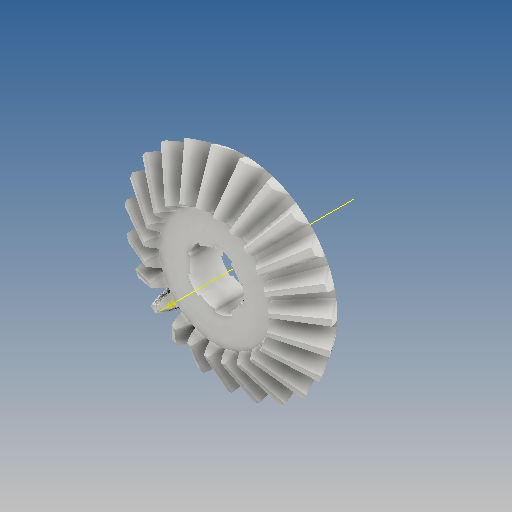
# Autodesk Inventor part: PWTR-0058
Saved by Autodesk Inventor 2021.1 (Build 251245000, 245)
## iProperties
CustomPartVersion: 1
Created: 2020-08-27
Material: Steel, Mild
Document SubType Name: Modeling
Designer: alid
Categories: <?xml version="1.0" encoding="UTF-16"?> <MemberInstance><Categories><FamilyTemplate><FamilyTemplateParameter ValueType="xs:double" Id="1" ObjectReferenceKey="da_z" ObjectType="kUserParameterObject"/><FamilyTemplateParameter ValueType="xs:double" Id="2" ObjectReferenceKey="da_b" ObjectType="kUserParameterObject"/><FamilyTemplateParameter ValueType="xs:double" Id="3" ObjectReferenceKey="da_beta" ObjectType="kUserParameterObject"/><FamilyTemplateParameter ValueType="xs:double" Id="4" ObjectReferenceKey="da_dae" ObjectType="kUserParameterObject"/><FamilyTemplateParameter ValueType="xs:double" Id="5" ObjectReferenceKey="da_ve" ObjectType="kUserParameterObject"/><FamilyTemplateParameter ValueType="xs:double" Id="6" ObjectReferenceKey="da_omega" ObjectType="kUserParameterObject"/><FamilyTemplateParameter ValueType="xs:string" Id="7" ObjectReferenceKey="EAIAABAAAAAAHwAAAAAAAIAAAAAAAAAA" ObjectType="83914240" SubObjectId="SurfaceGeometry"/></FamilyTemplate><ParamToTemplateMap><ParamToTemplate CategoryParameter="//CategoryParameter[@InternalName='046C89C9-8512-4d59-83FE-43B91F4F132A']" TemplateParameter="1"/><ParamToTemplate CategoryParameter="//CategoryParameter[@InternalName='2552DF32-E462-4b46-AEBF-C6C7768E72AC']" TemplateParameter="2"/><ParamToTemplate CategoryParameter="//CategoryParameter[@InternalName='C9EE641D-15FC-4fae-A226-E94C4372FDD7']" TemplateParameter="3"/><ParamToTemplate><ParamToTemplate CategoryParameter="//CategoryParameter[@InternalName='00B6519A-459B-49c7-AD84-2E56D39A5744']" ConstantValue="0.000000"/></ParamToTemplate><ParamToTemplate><ParamToTemplate CategoryParameter="//CategoryParameter[@InternalName='04B31F0E-C7A6-4894-AA32-9629BEFACF47']" ConstantValue="1.000000"/></ParamToTemplate><ParamToTemplate><ParamToTemplate CategoryParameter="//CategoryParameter[@InternalName='43CBEC2E-7847-49e7-A936-2F7889FCB2D9']" ConstantValue="0.200000"/></ParamToTemplate><ParamToTemplate><ParamToTemplate CategoryParameter="//CategoryParameter[@InternalName='B1EFC894-105D-4ebd-86BF-FA20ED196853']" ConstantValue="0.266800"/></ParamToTemplate><ParamToTemplate><ParamToTemplate CategoryParameter="//CategoryParameter[@InternalName='51175063-3D10-4879-93E8-6246FE8B403D']" ConstantValue="2060000000.000000"/></ParamToTemplate><ParamToTemplate><ParamToTemplate CategoryParameter="//CategoryParameter[@InternalName='A3A52E27-4454-46a9-B0BD-C932399B70AF']" ConstantValue="0.300000"/></ParamToTemplate><ParamToTemplate CategoryParameter="//CategoryParameter[@InternalName='2A200944-5A8C-41ca-B96E-8520D2E510F1']" TemplateParameter="4"/><ParamToTemplate><ParamToTemplate CategoryParameter="//CategoryParameter[@InternalName='1A637F62-92C8-44bc-B81F-10802510B579']" ConstantValue="4.349894"/></ParamToTemplate><ParamToTemplate CategoryParameter="//CategoryParameter[@InternalName='B52DD4BE-6863-48fb-BF58-89EF6F9EC65C']" TemplateParameter="5"/><ParamToTemplate><ParamToTemplate CategoryParameter="//CategoryParameter[@InternalName='3956BFF2-84D2-457d-93C2-9B0613DEBA67']" ConstantValue="1.202891"/></ParamToTemplate><ParamToTemplate CategoryParameter="//CategoryParameter[@InternalName='739CFA02-461B-4bf8-8049-181FCAD8B28F']" TemplateParameter="6"/><ParamToTemplate><ParamToTemplate CategoryParameter="//CategoryParameter[@InternalName='A27E999F-E2CE-4481-8A2A-EBF499C4C3C5']" ConstantValue="0.000000"/></ParamToTemplate><ParamToTemplate><ParamToTemplate CategoryParameter="//CategoryParameter[@InternalName='9E1B4470-B2D3-4ff1-B813-535BB4CDF51A']" ConstantValue="3520000.000000"/></ParamToTemplate><ParamToTemplate><ParamToTemplate CategoryParameter="//CategoryParameter[@InternalName='F8452263-BFF6-458c-9FB1-07C4B99E95CD']" ConstantValue="11400000.000000"/></ParamToTemplate><ParamToTemplate><ParamToTemplate CategoryParameter="//CategoryParameter[@InternalName='3E3BB259-FD49-497f-8171-6EBC954A3479']" ConstantValue="2.000000"/></ParamToTemplate><ParamToTemplate CategoryParameter="//CategoryParameter[@InternalName='27C3BAF2-7550-4e4b-AE2C-0DB134B7D9B7']" TemplateParameter="7"/></ParamToTemplateMap><Category DisplayName="Gear" InternalName="DC85795E-93AB-48d5-8EEE-5A27447B64BD" Mnemonic="Gear"><CategoryParameter DisplayName="z" InternalName="046C89C9-8512-4d59-83FE-43B91F4F132A" Mnemonic="z"/><CategoryParameter DisplayName="b" InternalName="2552DF32-E462-4b46-AEBF-C6C7768E72AC" Mnemonic="b"/><CategoryParameter DisplayName="||b|" InternalName="C9EE641D-15FC-4fae-A226-E94C4372FDD7" Mnemonic="beta"/><CategoryParameter DisplayName="x" InternalName="00B6519A-459B-49c7-AD84-2E56D39A5744" Mnemonic="x"/><CategoryParameter DisplayName="a*" InternalName="04B31F0E-C7A6-4894-AA32-9629BEFACF47" Mnemonic="a"/><CategoryParameter DisplayName="c*" InternalName="43CBEC2E-7847-49e7-A936-2F7889FCB2D9" Mnemonic="c"/><CategoryParameter DisplayName="r|.f|*" InternalName="B1EFC894-105D-4ebd-86BF-FA20ED196853" Mnemonic="rf"/><CategoryParameter DisplayName="E" InternalName="51175063-3D10-4879-93E8-6246FE8B403D" Mnemonic="E"/><CategoryParameter DisplayName="||m|" InternalName="A3A52E27-4454-46a9-B0BD-C932399B70AF" Mnemonic="mi"/><Category DisplayName="BevelGear" InternalName="0C98F69A-0C2B-4791-B2FE-7691BB227E77" Mnemonic="BevelGear"><CategoryParameter DisplayName="d|.ae|" InternalName="2A200944-5A8C-41ca-B96E-8520D2E510F1" Mnemonic="dae"/><CategoryParameter DisplayName="d|.ai|" InternalName="1A637F62-92C8-44bc-B81F-10802510B579" Mnemonic="dai"/><CategoryParameter DisplayName="A|.e|" InternalName="B52DD4BE-6863-48fb-BF58-89EF6F9EC65C" Mnemonic="ve"/><CategoryParameter DisplayName="A|.i|" InternalName="3956BFF2-84D2-457d-93C2-9B0613DEBA67" Mnemonic="vi"/><CategoryParameter DisplayName="||S|" InternalName="739CFA02-461B-4bf8-8049-181FCAD8B28F" Mnemonic="omega"/><CategoryParameter DisplayName="x|.t|" InternalName="A27E999F-E2CE-4481-8A2A-EBF499C4C3C5" Mnemonic="xt"/><CategoryParameter DisplayName="||s||.Flim|" InternalName="9E1B4470-B2D3-4ff1-B813-535BB4CDF51A" Mnemonic="sFlim"/><CategoryParameter DisplayName="||s||.Hlim|" InternalName="F8452263-BFF6-458c-9FB1-07C4B99E95CD" Mnemonic="sHlim"/><CategoryParameter DisplayName="type" InternalName="3E3BB259-FD49-497f-8171-6EBC954A3479" Mnemonic="type"/><CategoryParameter DisplayName="PitchDiameter" InternalName="27C3BAF2-7550-4e4b-AE2C-0DB134B7D9B7" Mnemonic="IDS_PITCHDIAM"/></Category></Category></Categories></MemberInstance>
Mass: 60.9118 g
Surface Area: 34.3074 cm^2
Volume: 7.7496 cm^3
Density: 7.86 g/cm^3
Appearance: Steel
Description: Bevel Transfer Gear
Part Number: PWTR-0058
Author: alid
Revision Number: A
Autodesk Inventor part; units mm, degrees
ref_plane "Mesh Plane2" through (0, 0, 0) normal (0.9906859, 0.1361666, 0) x (0, 0, 1)
sketch "Teeth Body Sketch" plane through (0, 0, 0) normal (1, 0, 0) x (0, 1, 0)
  line L0 (0, 0) -> (32.533436, -25.515398) construction
  line L1 (32.533436, -25.515398) -> (36.138803, -19.987168)
  line L2 (36.138803, -19.987168) -> (0, 0) construction
  line L3 (34.5, -22.5) -> (0, 0) construction
  line L4 (19.579646, -15.35597) -> (21.74947, -12.028907)
  line L5 (32.533436, -25.515398) -> (19.579646, -15.35597)
  line L6 (36.138803, -19.987168) -> (21.74947, -12.028907)
  line L7 (0, -24.879989) -> (0, 4.146665)
  line L8 (0, -22.5) -> (36.138803, -22.5) construction
  dimension "d0" = 69
  dimension "d1" = 65.06687
  dimension "d2" = 72.27761
  dimension "d3" = 16.4
  dimension "d4" = 19.98717
  constraints: 16 end point, 4 point on line, 3 perpendicular, 2 collinear, 1 horizontal alignment, 1 vertical alignment
  measures "d0" diameter of L3.start L7
  measures "d1" diameter of L0.end L7
  measures "d2" diameter of L1.end L7
  measures "d3" distance between parallel lines of L1 L4
  measures "d4" vertical distance of L1.end L0.start
revolve "Teeth Body" add sketch "Teeth Body Sketch" angle 360 about axis through (0, 0, 0) along (0, 0, 1)
ref_plane "Tooth Plane" through (0, 34.5, -22.5) normal (0, -0.8376106, 0.5462678) x (1, 0, 0)
sketch "Start Sketch" plane through (0, 34.5, -22.5) normal (0, -0.8376106, 0.5462678) x (1, 0, 0)
  line L0 (0, -39.723332) -> (0, 12.461154)
  arc A0 (-1.111235, -4.392) -> (-5.068702, 4.791205) centre (-23.36018, -8.535768) ccw
  arc A1 (5.068702, 4.791205) -> (1.111235, -4.392) centre (23.36018, -8.535768) ccw
  line L1 (-1.111235, -4.392) -> (1.111235, -4.392)
  arc A2 (5.068702, 4.791205) -> (-5.068702, 4.791205) centre (0, -63.155839) ccw
  dimension "d7" = 22.63154
  dimension "d8" = 23.36018
  dimension "d9" = 54.62007
  dimension "d57" = 68.13584
  dimension "d58" = 58.76384
  constraints: 6 point on circle, 3 centre point, 3 symmetric about line, 2 end point, 1 coincident, 1 perpendicular, 1 other
  measures "d7" radius of A0
  measures "d8" horizontal distance of point (0, -63.156) A0.centre
  measures "d9" vertical distance of point (0, -63.156) A0.centre
  measures "d57" radius of A2
  measures "d58" distance from line of A2.centre L1
sketch "End Sketch" plane through (0, 20.486775, -13.36094) normal (0, -0.8376106, 0.5462678) x (1, 0, 0)
  line L0 (0, -23.451185) -> (0, 7.356604)
  arc A0 (-0.659873, -2.608055) -> (-3.009894, 2.845111) centre (-13.871732, -5.068706) ccw
  arc A1 (3.009894, 2.845111) -> (0.659873, -2.608055) centre (13.871732, -5.068706) ccw
  line L1 (-0.659873, -2.608055) -> (0.659873, -2.608055)
  arc A2 (3.009894, 2.845111) -> (-3.009894, 2.845111) centre (0, -37.503172) ccw
  dimension "d12" = 13.43905
  dimension "d15" = 13.87173
  dimension "d16" = 32.43447
  dimension "d59" = 40.46039
  dimension "d60" = 34.89512
  constraints: 6 point on circle, 3 centre point, 3 symmetric about line, 2 end point, 1 coincident, 1 other
  measures "d12" radius of A0
  measures "d15" horizontal distance of A0.centre point (0, -37.503)
  measures "d16" vertical distance of A0.centre point (0, -37.503)
  measures "d59" radius of A2
  measures "d60" distance from line of A2.centre L1
loft "Loft" cut profiles "Start Sketch", "End Sketch"
pattern_circular "Circular Pattern" count 23 over 360 about axis through (0, 0, 0) along (0, 0, 1) of "Loft"
ref_plane "End Plane" through (0, 20.486775, -13.36094) normal (0, -0.8376106, 0.5462678) x (1, 0, 0)
sketch3d "3D Sketch Right"
ref_plane "End Plane Right" through (-4.87651, 19.897929, -13.36094) normal (0.1993782, -0.8135354, 0.5462678) x (0.9712573, 0.2380321, 0)
sketch "End Sketch Right" plane through (-4.87651, 19.897929, -13.36094) normal (0.1993782, -0.8135354, 0.5462678) x (0.9712573, 0.2380321, 0)
  arc A0 (-0.659873, -2.608055) -> (-3.009894, 2.845111) centre (-13.871732, -5.068706) ccw
  line L0 (0, -48.37326) -> (0, 13.825579)
  arc A1 (3.009894, 2.845111) -> (0.659873, -2.608055) centre (13.871732, -5.068706) ccw
  line L1 (-0.659873, -2.608055) -> (0.659873, -2.608055)
  arc A2 (3.009894, 2.845111) -> (-3.009894, 2.845111) centre (0, -37.503172) ccw
  dimension "d70" = 13.87173
  dimension "d71" = 32.43447
  dimension "d72" = 13.43905
  dimension "d73" = 34.89512
  dimension "d74" = 40.46039
  constraints: 6 point on circle, 3 centre point, 3 symmetric about line, 2 end point, 1 coincident, 1 perpendicular, 1 other
  measures "d70" horizontal distance of A2.centre A0.centre
  measures "d71" vertical distance of point (0, -37.503) A0.centre
  measures "d72" radius of A0
  measures "d73" distance from line of point (0, -37.503) L1
  measures "d74" radius of A2
feature "Loft Right" [suppressed]
pattern_circular "Circular Pattern Right" [suppressed]
sketch3d "3D Sketch Left"
ref_plane "End Plane Left" through (4.872543, 19.897929, -13.358824) normal (-0.1992319, -0.8136001, 0.5462247) x (0.971302, -0.2378494, 0)
sketch "End Sketch Left" plane through (4.872543, 19.897929, -13.358824) normal (-0.1992319, -0.8136001, 0.5462247) x (0.971302, -0.2378494, 0)
  line L0 (0, -50.480896) -> (0, 15.931763)
  arc A0 (-0.659873, -2.609312) -> (-3.009894, 2.843855) centre (-13.871732, -5.069962) ccw
  arc A1 (3.009894, 2.843855) -> (0.659873, -2.609312) centre (13.871732, -5.069962) ccw
  line L1 (-0.659873, -2.609312) -> (0.659873, -2.609312)
  ellipse E0 centre (0, -10.075878) end of major axis (21.74947, -10.075878) minor radius 11.880098
  arc A2 (3.009894, 2.843855) -> (-3.009894, 2.843855) centre (0, -37.504429) ccw
  dimension "d56" = 11.8801
  dimension "d30" = 13.43905
  dimension "d31" = 13.87173
  dimension "d32" = 32.43447
  dimension "d61" = 40.46039
  dimension "d62" = 34.89512
  constraints: 6 point on circle, 3 centre point, 3 symmetric about line, 2 end point, 1 coincident, 2 other
  measures "d30" radius of A0
  measures "d31" horizontal distance of point (0, -37.504) A0.centre
  measures "d32" vertical distance of A0.centre point (0, -37.504)
  measures "d61" radius of A2
  measures "d62" distance from line of point (0, -37.504) L1
feature "Loft Left" [suppressed]
pattern_circular "Circular Pattern Left" [suppressed]
sketch "Body Sketch" plane through (0, 0, 0) normal (1, 0, 0) x (0, 1, 0)
  line L0 (0, -22.382477) -> (0, -10.838407)
  line L1 (32.533436, -25.515398) -> (19.579646, -15.35597)
  line L2 (19.579646, -15.35597) -> (0, -15.35597)
  line L3 (32.533436, -25.515398) -> (0, -25.515398)
  constraints: 4 end point, 2 perpendicular, 2 point on line
sketch "Body Sketch outline for Fix Body" plane through (0, 0, 0) normal (1, 0, 0) x (0, 1, 0)
  line L0 (0, -25.515398) -> (32.533436, -25.515398)
  line L1 (0, -15.35597) -> (0, -25.515398)
  line L2 (19.579646, -15.35597) -> (0, -15.35597)
  line L3 (32.533436, -25.515398) -> (19.579646, -15.35597)
revolve "Fix Body" add sketch "Body Sketch outline for Fix Body" angle 360 about axis through (0, 0, 0) along (0, 0, 1)
sketch "Sketch6" plane through (0, 0, 0) normal (1, 0, 0) x (0, 1, 0)
  line L0 (34.5, -22.5) -> (0, 0) projected
  line L1 (0, -21.6) -> (0, 3.6) projected
surface revolve "Pitch Diameter" sketch "Sketch6" angle 360 about axis through (0, 0, 0) along (0, 0, 1) shown no curves L0
sketch "Sketch8" plane through (0, 0, -25.515398) normal (0, 0, -1) x (-1, 0, 0)
  circle A0 centre (0, 0) radius 17
  circle A1 centre (0, 0) radius 9
  circle A2 centre (0, 0) radius 10
  line L0 (9.510565, 3.09017) -> (8.45286, 3.09017) construction
  line L1 (9.510565, -3.09017) -> (8.45286, -3.09017) construction
  line L2 (0, 0) -> (10, 0) construction
  line L3 (9.510565, -3.09017) -> (0, 0)
  line L4 (9.510565, 3.09017) -> (0, 0)
  point P0 (8.559509, 2.781153)
  point P1 (8.559509, -2.781153)
  dimension "d94" = 34
  dimension "d100" = 18
  dimension "d103" = 20
  dimension "d110" = 36
  constraints: 10 end point, 5 point on circle, 3 centre point, 3 coincident, 2 parallel, 1 horizontal, 1 other
  measures "d94" diameter of A0
  measures "d100" diameter of A1
  measures "d103" diameter of A2
  measures "d110" angle of L3 L4
extrude "Extrusion1" add sketch "Sketch8" along normal blind 1.303 contours A0 | A1 L4 A2 L3 | A1 L3 A2 L4
extrude "Extrusion2" cut sketch "Sketch8" against normal through all both and the other way through all contours A1 L3 L4 | A1 L4 A2 L3 | L4 L3 A1 | A1 L3 A2 L4
extrude "Extrusion3" add sketch "Sketch8" against normal up to surface (11.462428 mm away) from surface at 1.303 contours A1 L4 A2 L3 picked at (9.648406, -0.348428)
pattern_circular "Circular Pattern4" count 5 over 360 about axis through (0, 0, 0) along (0, 0, 1) of "Extrusion3"
equation "\"d0\" = da_de"
equation "\"d1\" = da_dfe"
equation "\"d2\" = da_dae"
equation "\"d3\" = da_b"
equation "\"d4\" = da_ve"
equation "\"d7\" = fd_rr"
equation "\"d8\" = fd_x"
equation "\"d9\" = fd_y"
equation "\"d57\" = 0.5 * fd_dva + 0.3 * da_he"
equation "\"d58\" = 0.5 * fd_dva - 1.12 * da_he"
equation "\"da_teethtype\" = 0"
equation "\"da_b\" = 16.4"
equation "\"da_de\" = 69"
equation "\"da_dae\" = 72.27761"
equation "\"da_dfe\" = 65.06687"
equation "\"da_le\" = 41.18859"
equation "\"da_omega\" = 90deg"
equation "\"da_beta\" = 0"
equation "\"da_delta\" = 56.888658deg"
equation "\"da_alpha\" = 20deg"
equation "\"da_he\" = 6.6"
equation "\"da_ve\" = 19.98717"
equation "\"da_zv\" = 42.103893"
equation "\"fd_loft\" = da_b + 0.05 * da_he"
equation "\"fd_x\" = fd_x1 + fd_x2"
equation "\"fd_y\" = fd_y1 - fd_y2"
equation "\"fd_dd\" = fd_dva - 0.8 * da_he"
equation "\"da_dvw\" = 126.31168"
equation "\"d11\" = fd_loft"
equation "\"da_dm\" = 55.26319"
equation "\"da_x\" = 0"
equation "\"da_m\" = 3"
equation "\"d50\" = da_omega"
equation "\"fd_rr\" = 22.631535"
equation "\"fd_dva\" = 132.311678"
equation "\"fd_x1\" = 2.381809"
equation "\"fd_x2\" = 20.978371"
equation "\"fd_y1\" = 63.11091"
equation "\"fd_y2\" = 8.490839"
body "Solid1"
body "Srf1"
